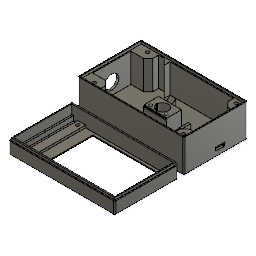
Wärmebildkamera-Gehäuse-v49 (Autodesk Fusion 360 design; units mm, degrees)
Autodesk Fusion 360 part; units mm, degrees
box "Grundkörper Quader1" add length 55 width 92 height 11 placed x (0, 0, 1) y (1, 0, 0) z (0, 1, 0) at (-92, 0, 0) makes body 1
box "Grundkörper Quader3" cut length 51 width 83 height -6 placed x (0, 0, -1) y (-1, 0, 0) z (0, 1, 0) at (-2, 11, 53) bodies 1
box "Grundkörper Quader4" cut length 45.9499 width 60 height -6 placed x (0, 0, -1) y (-1, 0, 0) z (0, 1, 0) at (-9.4927, 5, 50.5086) bodies 1
box "Grundkörper Quader5" cut length 51 width 82 height -4 placed x (0, 0, -1) y (-1, 0, 0) z (0, 1, 0) at (-8, 5, 53) bodies 1
sketch "Skizze11" plane through (0, 11, 0) normal (0, 1, 0) x (-1, 0, 0)
  line L0 (2, 53) -> (85, 53)
  line L1 (85, 53) -> (85, 2)
  line L2 (85, 2) -> (2, 2)
  line L3 (2, 2) -> (2, 53)
  line L4 (0, 0) -> (92, 0)
  line L5 (92, 0) -> (92, 55)
  line L6 (92, 55) -> (0, 55)
  line L7 (0, 55) -> (0, 0)
  line L8 (85, 53) -> (90, 53)
  line L9 (90, 53) -> (90, 2)
  line L10 (90, 2) -> (85, 2)
  line L11 (85, 2) -> (85, 53)
extrude "Extrusion1" cut sketch "Skizze11" against normal blind 4 contours L1 L8 L9 L10 L11 bodies 1
sketch "Skizze15" plane through (0, 11, 0) normal (0, 1, 0) x (-1, 0, 0)
  line L0 (2, 53) -> (90, 53)
  line L1 (90, 53) -> (90, 2)
  line L2 (90, 2) -> (2, 2)
  line L3 (2, 2) -> (2, 53)
  line L4 (0, 0) -> (92, 0)
  line L5 (92, 0) -> (92, 55)
  line L6 (92, 55) -> (0, 55)
  line L7 (0, 55) -> (0, 0)
  line L8 (91, 1) -> (1, 1)
  line L9 (1, 1) -> (1, 54)
  line L10 (1, 54) -> (91, 54)
  line L11 (91, 54) -> (91, 1)
extrude "Extrusion3" add sketch "Skizze15" along normal blind 2 contours L8 L9 L10 L11 bodies 1
sketch "Skizze16" plane through (0, 0, 0) normal (0, 1, 0) x (1, 0, 0)
  line L0 (0, 5) -> (-92, 5)
  line L1 (-92, 5) -> (-92, 60)
  line L2 (-92, 60) -> (0, 60)
  line L3 (0, 60) -> (0, 5)
extrude "Extrusion4" add sketch "Skizze16" along normal blind 2 separate body makes body 2
sketch "Skizze17" plane through (0, 2, 0) normal (0, 1, 0) x (-1, 0, 0)
  line L0 (0, -60) -> (92, -60)
  line L1 (92, -60) -> (92, -5)
  line L2 (92, -5) -> (0, -5)
  line L3 (0, -5) -> (0, -60)
  line L4 (90, -58) -> (2, -58)
  line L5 (2, -58) -> (2, -7)
  line L6 (2, -7) -> (90, -7)
  line L7 (90, -7) -> (90, -58)
extrude "Extrusion5" add sketch "Skizze17" along normal blind 25 bodies 2
sketch "Skizze18" plane through (0, 27, 0) normal (0, 1, 0) x (-1, 0, 0)
  line L0 (2, -7) -> (90, -7)
  line L1 (90, -7) -> (90, -58)
  line L2 (90, -58) -> (2, -58)
  line L3 (2, -58) -> (2, -7)
  line L4 (0, -5) -> (0, -60)
  line L5 (0, -60) -> (92, -60)
  line L6 (92, -60) -> (92, -5)
  line L7 (92, -5) -> (0, -5)
  line L8 (91, -59) -> (1, -59)
  line L9 (1, -59) -> (1, -6)
  line L10 (1, -6) -> (91, -6)
  line L11 (91, -6) -> (91, -59)
extrude "Extrusion6" add sketch "Skizze18" along normal blind 2 contours L4 L5 L6 L7 bodies 2
sketch "Skizze19" plane through (0, 2, 0) normal (0, 1, 0) x (-1, 0, 0)
  line L0 (2, -7) -> (2, -58)
  line L1 (2, -58) -> (90, -58)
  line L2 (90, -58) -> (90, -7)
  line L3 (90, -7) -> (2, -7)
  line L4 (10, -7) -> (75, -7)
  line L5 (75, -7) -> (75, -26.5)
  line L6 (75, -26.5) -> (10, -26.5)
  line L7 (10, -26.5) -> (10, -7)
  dimension "d50" = 65
  dimension "d51" = 19.5
extrude "Extrusion7" add sketch "Skizze19" along normal blind 12 contours L3 L4 L5 L6 L7 bodies 2
sketch "Skizze20" plane through (-75, 0, 0) normal (-1, 0, 0) x (0, 0, 1)
  line L0 (-26.5, 2) -> (-7, 2)
  line L1 (-7, 2) -> (-7, 14)
  line L2 (-7, 14) -> (-26.5, 14)
  line L3 (-26.5, 14) -> (-26.5, 2)
  circle A0 centre (-16.75, 11.25) radius 9.25
  dimension "d54" = 18.5
  measures "d54" diameter of A0
extrude "Extrusion8" cut sketch "Skizze20" against normal blind 65 contours L2 A0 picked at (-17.65, 9.3946) bodies 2
sketch "Skizze21" plane through (0, 2, 0) normal (0, 1, 0) x (-1, 0, 0)
  line L0 (75, -7) -> (75, -16.75)
  line L1 (75, -16.75) -> (75, -26.5)
  line L2 (75, -26.5) -> (10, -26.5)
  line L3 (10, -26.5) -> (10, -16.75)
  line L4 (10, -16.75) -> (10, -7)
  line L5 (10, -7) -> (2, -7)
  line L6 (2, -7) -> (2, -58)
  line L7 (2, -58) -> (90, -58)
  line L8 (90, -58) -> (90, -7)
  line L9 (90, -7) -> (75, -7)
  circle A0 centre (46, -32.5) radius 4.75
  line L10 (56.0142, -26.5) -> (36, -26.5)
  line L11 (36, -26.5) -> (36, -39)
  line L12 (36, -39) -> (56.0142, -39)
  line L13 (56.0142, -39) -> (56.0142, -26.5)
  dimension "d57" = 9.5
  measures "d57" diameter of A0
extrude "Extrusion9" add sketch "Skizze21" along normal blind 13 contours L2 L10 L11 L12 L13 bodies 2
extrude "Extrusion10" cut 1 faces at (-47.2238, 2, -31.2621) along direction (0, -1, 0) blind 2 on bodies 2 bodies 2
sketch "Skizze22" plane through (0, 15, 0) normal (0, 1, 0) x (-1, 0, 0)
  circle A0 centre (46, -32.5) radius 4.75
  line L0 (56.0142, -39) -> (56.0142, -26.5)
  line L1 (56.0142, -26.5) -> (36, -26.5)
  line L2 (36, -26.5) -> (36, -39)
  line L3 (36, -39) -> (56.0142, -39)
  line L4 (51.5, -33) -> (50.5, -33)
  line L5 (50.5, -33) -> (50.5, -32)
  line L6 (50.5, -32) -> (51.5, -32)
  line L7 (51.5, -32) -> (51.5, -33)
extrude "Extrusion11" cut sketch "Skizze22" against normal blind 5 contours A0 L4 L6 L7 bodies 2
sketch "Skizze24" plane through (0, 2, 0) normal (0, 1, 0) x (-1, 0, 0)
  line L0 (56.0142, -26.5) -> (56.0142, -39)
  line L1 (56.0142, -39) -> (36, -39)
  line L2 (36, -39) -> (36, -26.5)
  line L3 (36, -26.5) -> (10, -26.5)
  line L4 (10, -26.5) -> (10, -16.75)
  line L5 (10, -16.75) -> (10, -7)
  line L6 (10, -7) -> (2, -7)
  line L7 (2, -7) -> (2, -58)
  line L8 (2, -58) -> (90, -58)
  line L9 (90, -58) -> (90, -7)
  line L10 (90, -7) -> (75, -7)
  line L11 (75, -7) -> (75, -16.75)
  line L12 (75, -16.75) -> (75, -26.5)
  line L13 (75, -26.5) -> (56.0142, -26.5)
  line L14 (82, -58) -> (90, -58)
  line L15 (90, -58) -> (90, -49)
  line L16 (90, -49) -> (82, -49)
  line L17 (82, -49) -> (82, -58)
  line L18 (90, -16) -> (82, -16)
  line L19 (82, -16) -> (82, -7)
  line L20 (82, -7) -> (90, -7)
  line L21 (90, -7) -> (90, -16)
  line L22 (2, -58) -> (10, -58)
  line L23 (10, -58) -> (10, -49)
  line L24 (10, -49) -> (2, -49)
  line L25 (2, -49) -> (2, -58)
  line L26 (2, -7) -> (10, -7)
  line L27 (10, -7) -> (10, -16)
  line L28 (10, -16) -> (2, -16)
  line L29 (2, -16) -> (2, -7)
extrude "Extrusion13" add sketch "Skizze24" along normal blind 27 contours L9 L10 L18 L19 L20 L21 | L5 L6 L7 L26 L27 L28 L29 | L8 L9 L14 L15 L16 L17 | L7 L8 L22 L23 L24 L25 bodies 2
sketch "Skizze25" plane through (0, 29, 0) normal (0, 1, 0) x (-1, 0, 0)
  line L0 (90, -7) -> (82, -7)
  line L1 (82, -7) -> (82, -16)
  line L2 (82, -16) -> (90, -16)
  line L3 (90, -16) -> (90, -7)
  circle A0 centre (5, -55.5) radius 1.5
  circle A1 centre (5, -9.5) radius 1.5
  dimension "d72" = 3
  dimension "d73" = 3
  measures "d72" diameter of A0
  measures "d73" diameter of A1
extrude "Extrusion14" cut sketch "Skizze25" against normal blind 25 contours A0 | A1 bodies 2
extrude "Extrusion15" cut 4 faces at (-84.6667, 29, -52) (-84.6667, 29, -10) (-5.7779, 29, -14.3208) (-5.7779, 29, -50.6792) along direction (0, -1, 0) blind 7 on bodies 2 bodies 2
delete_face "Fläche löschen1" 1 faces at (-50.6361, 8.3333, -33.5338) on bodies 2
sketch "Skizze26" plane through (0, 15, 0) normal (0, 1, 0) x (-1, 0, 0)
  line L0 (36, -26.5) -> (36, -39)
  line L1 (36, -39) -> (56.0142, -39)
  line L2 (56.0142, -39) -> (56.0142, -26.5)
  line L3 (56.0142, -26.5) -> (36, -26.5)
  circle A0 centre (46.0071, -32.5) radius 5
  circle A1 centre (39.2493, -29) radius 1.5
  circle A2 centre (52.7493, -29) radius 1.5
  line L4 (51.5, -33) -> (50.9821, -33)
  line L5 (51.5, -33) -> (51.5, -32)
  line L6 (51.5, -32) -> (50.9821, -32)
  line L7 (46.0088, -27.5) -> (52.7588, -27.5022)
  dimension "d78" = 10
  dimension "d81" = 3
  dimension "d82" = 3
  dimension "d87" = 6.75
  measures "d78" diameter of A0
  measures "d81" diameter of A1
  measures "d82" diameter of A2
extrude "Extrusion16" cut sketch "Skizze26" against normal blind 15 contours A0 bodies 2
extrude "Extrusion17" cut sketch "Skizze26" against normal blind 13 contours A1 | A2 bodies 2
thread "Gewinde5" "ISO Metric profile 3.0 M3x0.5 6H" major diameter 3.086 minor diameter 2.529 pitch 0.5 angle 60 resizes the face on face at (-52.1324, 6.3333, -30.3673) on bodies 2
thread "Gewinde6" "ISO Metric profile 3.0 M3x0.5 6H" major diameter 3.086 minor diameter 2.529 pitch 0.5 angle 60 resizes the face on face at (-38.565, 10.6667, -30.3348) on bodies 2
move_face "Fläche verschieben1" by (-1, 0, 0) 1 faces at (-9.4927, 0.3333, 35.1919) on bodies 1
extrude "Extrusion18" cut sketch "Skizze26" against normal blind 6 contours A0 L4 L5 L6 bodies 2
fillet "Abrundung1" radius 1 1 edges at (0, 14.5, -60) on bodies 2
fillet "Abrundung2" radius 1 1 edges at (0, 14.5, -5) on bodies 2
fillet "Abrundung3" radius 1 5 edges at (-46.5, 0, -60) (-0.2929, 0, -59.7071) (0, 0, -32.5) (-0.2929, 0, -5.2929) (-46.5, 0, -5) on bodies 2
fillet "Abrundung4" radius 1 5 edges at (-92, 15, -5) (-92, 0.2929, -5.2929) (-92, 0, -32.5) (-92, 0.2929, -59.7071) (-92, 15, -60) on bodies 2
fillet "Abrundung5" radius 1 1 edges at (0, 0, 27.5) on bodies 1
fillet "Abrundung6" radius 1 3 edges at (0, 6, 55) (-0.2929, 0.2929, 55) (-46.5, 0, 55) on bodies 1
fillet "Abrundung7" radius 1 3 edges at (0, 6, 0) (-0.2929, 0.2929, 0) (-46.5, 0, 0) on bodies 1
fillet "Abrundung8" radius 1 5 edges at (-92, 6, 55) (-92, 0.2929, 54.7071) (-92, 0, 27.5) (-92, 0.2929, 0.2929) (-92, 6, 0) on bodies 1
sketch "Skizze27" plane through (0, 2, 0) normal (0, 1, 0) x (-1, 0, 0)
  line L0 (82, -58) -> (82, -49)
  line L1 (82, -49) -> (90, -49)
  line L2 (90, -49) -> (90, -16)
  line L3 (90, -16) -> (82, -16)
  line L4 (82, -16) -> (82, -7)
  line L5 (82, -7) -> (75, -7)
  line L6 (75, -7) -> (75, -16.75)
  line L7 (75, -16.75) -> (75, -26.5)
  line L8 (75, -26.5) -> (56.0142, -26.5)
  line L9 (56.0142, -26.5) -> (56.0142, -39)
  line L10 (56.0142, -39) -> (36, -39)
  line L11 (36, -39) -> (36, -26.5)
  line L12 (36, -26.5) -> (10, -26.5)
  line L13 (10, -26.5) -> (10, -16.75)
  line L14 (10, -16.75) -> (10, -16)
  line L15 (10, -16) -> (2, -16)
  line L16 (2, -16) -> (2, -49)
  line L17 (2, -49) -> (10, -49)
  line L18 (10, -49) -> (10, -58)
  line L19 (10, -58) -> (82, -58)
  line L20 (2, -28) -> (28, -28)
  line L21 (28, -28) -> (28, -45)
  line L22 (28, -45) -> (2, -45)
  line L23 (2, -45) -> (2, -28)
  line L24 (7, -44) -> (23, -44)
  line L25 (23, -44) -> (23, -48)
  line L26 (23, -48) -> (7, -48)
  line L27 (7, -48) -> (7, -44)
  line L28 (7, -29) -> (23, -29)
  line L29 (23, -29) -> (23, -26.5)
  line L30 (23, -26.5) -> (7, -26.5)
  line L31 (7, -26.5) -> (7, -29)
  dimension "d98" = 26
  dimension "d99" = 17
  measures "d98" distance of origin
extrude "Extrusion19" add sketch "Skizze27" along normal blind 5 contours L22 L24 L25 L27 | L22 L25 L26 L27 | L12 L20 L29 L30 L31 | L20 L28 L29 L31 bodies 2
sketch "Skizze28" plane through (-23, 0, 0) normal (-1, 0, 0) x (0, 0, 1)
  line L0 (-48, 2) -> (-44, 2)
  line L1 (-44, 2) -> (-44, 7)
  line L2 (-44, 7) -> (-48, 7)
  line L3 (-48, 7) -> (-48, 2)
  line L4 (-44, 4) -> (-45.3671, 4)
  line L5 (-45.3671, 4) -> (-45.3671, 22.3058)
  line L6 (-45.3671, 22.3058) -> (-45.3907, 7)
  line L7 (-45.4065, 7) -> (-45.3907, 7)
  line L8 (-46, 7) -> (-48, 2)
  line L9 (-29, 2) -> (-29, 7)
  line L10 (-29, 4) -> (-28, 4)
  line L11 (-28, 4) -> (-28, 5)
  line L12 (-28, 5) -> (-29, 6)
  line L13 (-26.5, 7) -> (-29, 7)
  line L14 (-29, 6) -> (-28, 7)
extrude "Extrusion20" cut sketch "Skizze28" against normal blind 17 contours L2 L3 L8 | L1 L2 L4 L5 | L9 L10 L11 L12 bodies 2
sketch "Skizze29" plane through (-2, 0, 0) normal (-1, 0, 0) x (0, 0, 1)
  line L0 (-49, 22) -> (-49, 2)
  line L1 (-49, 2) -> (-16, 2)
  line L2 (-16, 2) -> (-16, 22)
  line L3 (-16, 22) -> (-7, 22)
  line L4 (-45.3671, 4) -> (-28, 4)
  line L5 (-28, 4) -> (-28, 5)
  line L6 (-28, 5) -> (-45.3671, 5)
  line L7 (-45.3671, 5) -> (-45.3671, 4)
  line L8 (-36.6835, 5) -> (-32.5, 5)
  line L9 (-32.5, 5) -> (-32.5, 8)
  line L10 (-32.5, 8) -> (-36.6835, 8)
  line L11 (-36.6835, 8) -> (-36.6835, 5)
  line L12 (-32.5, 8) -> (-40.5, 8)
  line L13 (-40.5, 8) -> (-40.5, 5)
  line L14 (-40.5, 5) -> (-32.5, 5)
  line L15 (-32.5, 5) -> (-32.5, 8)
  line L16 (-7, 22) -> (-7, 27)
  line L17 (-7, 27) -> (-58, 27)
  line L18 (-58, 27) -> (-58, 22)
  line L19 (-58, 22) -> (-49, 22)
extrude "Extrusion21" cut sketch "Skizze29" against normal blind 11 contours L6 L11 L12 L13 L14 | L6 L8 L9 L10 L11 L12 L14 L15 bodies 2
sketch "Skizze30" plane through (0, 2, 0) normal (0, 1, 0) x (-1, 0, 0)
  line L0 (23, -26.5) -> (23, -29)
  line L1 (23, -29) -> (7, -29)
  line L2 (7, -29) -> (7, -26.5)
  line L3 (10, -16.75) -> (10, -16)
  line L4 (10, -16) -> (2, -16)
  line L5 (2, -16) -> (2, -49)
  line L6 (2, -49) -> (10, -49)
  line L7 (10, -49) -> (10, -58)
  line L8 (10, -58) -> (82, -58)
  line L9 (82, -58) -> (82, -49)
  line L10 (82, -49) -> (90, -49)
  line L11 (90, -49) -> (90, -16)
  line L12 (90, -16) -> (82, -16)
  line L13 (82, -16) -> (82, -7)
  line L14 (82, -7) -> (75, -7)
  line L15 (75, -7) -> (75, -16.75)
  line L16 (75, -16.75) -> (75, -26.5)
  line L17 (75, -26.5) -> (56.0142, -26.5)
  line L18 (56.0142, -26.5) -> (56.0142, -39)
  line L19 (56.0142, -39) -> (36, -39)
  line L20 (36, -39) -> (36, -26.5)
  line L21 (36, -26.5) -> (23, -26.5)
  line L22 (7, -48) -> (7, -44)
  line L23 (7, -44) -> (23, -44)
  line L24 (23, -44) -> (23, -48)
  line L25 (23, -48) -> (7, -48)
  line L26 (2, -32.5) -> (2, -40.5)
  line L27 (2, -36.5) -> (28.5, -36.5)
  line L28 (29.5, -40.4445) -> (33.5, -40.4445)
  line L29 (33.5, -40.4445) -> (33.5, -32.4445)
  line L30 (33.5, -32.4445) -> (29.5, -32.4445)
  line L31 (29.5, -32.4445) -> (29.5, -40.4445)
  line L32 (7, -26.5) -> (10, -26.5)
  line L33 (10, -26.5) -> (10, -16.75)
  dimension "d107" = 26.5
  measures "d107" distance of origin
extrude "Extrusion22" add sketch "Skizze30" along normal blind 5 contours L28 L29 L30 L31 bodies 2
sketch "Skizze31" plane through (0, 0, -26.5) normal (0, 0, -1) x (-1, 0, 0)
  line L0 (10, 7) -> (23, 7)
  line L1 (23, 7) -> (23, 2)
  line L2 (23, 2) -> (36, 2)
  line L3 (36, 2) -> (36, 14)
  line L4 (36, 14) -> (10, 14)
  line L5 (10, 14) -> (10, 7)
  line L6 (10, 7) -> (36, 7)
  line L7 (36, 7) -> (36, 14)
  line L8 (36, 14) -> (10, 14)
  line L9 (10, 14) -> (10, 7)
  line L10 (56.0142, 7) -> (75, 7)
  line L11 (75, 7) -> (75, 14)
  line L12 (75, 14) -> (56.0142, 14)
  line L13 (56.0142, 14) -> (56.0142, 7)
  line L14 (56.0142, 14) -> (56.0142, 2)
extrude "Extrusion23" cut sketch "Skizze31" against normal blind 4 contours L0 L3 L4 L5 L6 L7 L8 L9 | L10 L11 L12 L13 L14 bodies 2
sketch "Skizze32" plane through (0, 2, 0) normal (0, 1, 0) x (-1, 0, 0)
  line L0 (29.5, -32.4445) -> (33.5, -32.4445)
  line L1 (33.5, -32.4445) -> (33.5, -40.4445)
  line L2 (33.5, -40.4445) -> (29.5, -40.4445)
  line L3 (29.5, -40.4445) -> (29.5, -32.4445)
  line L4 (23, -26.5) -> (23, -29)
  line L5 (23, -29) -> (7, -29)
  line L6 (7, -29) -> (7, -26.5)
  line L7 (10, -16.75) -> (10, -16)
  line L8 (10, -16) -> (2, -16)
  line L9 (2, -16) -> (2, -49)
  line L10 (2, -49) -> (10, -49)
  line L11 (10, -49) -> (10, -58)
  line L12 (10, -58) -> (82, -58)
  line L13 (82, -58) -> (82, -49)
  line L14 (82, -49) -> (90, -49)
  line L15 (90, -49) -> (90, -16)
  line L16 (90, -16) -> (82, -16)
  line L17 (82, -16) -> (82, -7)
  line L18 (82, -7) -> (75, -7)
  line L19 (75, -7) -> (75, -16.75)
  line L20 (75, -16.75) -> (75, -26.5)
  line L21 (75, -26.5) -> (56.0142, -26.5)
  line L22 (56.0142, -26.5) -> (56.0142, -39)
  line L23 (56.0142, -39) -> (36, -39)
  line L24 (36, -39) -> (36, -26.5)
  line L25 (36, -26.5) -> (23, -26.5)
  line L26 (7, -48) -> (7, -44)
  line L27 (7, -44) -> (23, -44)
  line L28 (23, -44) -> (23, -48)
  line L29 (23, -48) -> (7, -48)
  line L30 (36, -39) -> (56, -39)
  line L31 (56, -39) -> (56, -39.7497)
  line L32 (56, -39.7497) -> (36, -39.7497)
  line L33 (36, -39.7497) -> (36, -39)
  line L34 (36, -58) -> (56, -58)
  line L35 (56, -58) -> (56, -56)
  line L36 (56, -56) -> (36, -56)
  line L37 (36, -56) -> (36, -58)
  line L38 (7, -26.5) -> (10, -26.5)
  line L39 (10, -26.5) -> (10, -16.75)
sketch "Skizze34" plane through (0, 0, -40.4445) normal (0, 0, -1) x (-1, 0, 0)
  line L0 (29.5, 2) -> (33.5, 2)
  line L1 (33.5, 2) -> (33.5, 7)
  line L2 (33.5, 7) -> (29.5, 7)
  line L3 (29.5, 7) -> (29.5, 2)
  line L4 (33.5, 2) -> (31.5, 7)
extrude "Extrusion27" cut sketch "Skizze34" against normal blind 9 contours L1 L2 L4 bodies 2
sketch "Skizze35" plane through (-92, 0, 0) normal (-1, 0, 0) x (0, 0, 1)
  line L0 (-6, 1) -> (-6, 29)
  line L1 (-6, 29) -> (-59, 29)
  line L2 (-59, 29) -> (-59, 1)
  line L3 (-59, 1) -> (-6, 1)
  circle A0 centre (-32.5, 12) radius 6
  dimension "d120" = 12
  measures "d120" diameter of A0
extrude "Extrusion28" cut sketch "Skizze35" against normal blind 30 contours A0 bodies 2
sketch "Skizze38" plane through (0, 27, 0) normal (0, 1, 0) x (-1, 0, 0)
  line L0 (1, -6) -> (1, -59)
  line L1 (1, -59) -> (91, -59)
  line L2 (91, -59) -> (91, -6)
  line L3 (91, -6) -> (1, -6)
  line L4 (2, -7) -> (90, -7)
  line L5 (90, -7) -> (90, -58)
  line L6 (90, -58) -> (2, -58)
  line L7 (2, -58) -> (2, -7)
chamfer "Fase2" distance 0.5 angle 45 1 edges at (-1, 5, -40.5) on bodies 2
chamfer "Fase3" distance 0.5 angle 45 1 edges at (-1, 5, -32.5) on bodies 2
extrude "Extrusion31" add 2 faces at (-31.6667, 9.6667, 2) (-88.3333, 9.6667, 2) along direction (0, 0, 1) blind 0.75 on bodies 1 bodies 1
extrude "Extrusion32" add 1 faces at (-31.6667, 8.3333, 53) along direction (0, 0, -1) blind 0.75 on bodies 1 bodies 1
extrude "Extrusion33" cut 1 faces at (-86.6667, 7, 19.25) along direction (0, -1, 0) blind 2 on bodies 1 bodies 1
extrude "Extrusion34" add 1 faces at (-8, 2.3333, 35.75) along direction (-1, 0, 0) blind 0.5 on bodies 1 bodies 1
sketch "Skizze40" plane through (0, 5, 0) normal (0, 1, 0) x (-1, 0, 0)
  line L0 (8.5, 52.25) -> (2, 52.25)
  line L1 (2, 52.25) -> (2, 2.75)
  line L2 (2, 2.75) -> (8.5, 2.75)
  line L3 (8.5, 2.75) -> (8.5, 52.25)
  circle A0 centre (5, 5.5) radius 1.5
  circle A1 centre (5, 49.5) radius 1.5
  dimension "d149" = 3
  dimension "d150" = 3
  measures "d149" diameter of A0
  measures "d150" diameter of A1
extrude "Extrusion35" cut sketch "Skizze40" against normal blind 26 contours A0 | A1 bodies 1
sketch "Skizze45" plane through (0, 1, 0) normal (0, 1, 0) x (-1, 0, 0)
  line L0 (8.5, 52.25) -> (8.5, 2.75)
  line L1 (8.5, 2.75) -> (90, 2.75)
  line L2 (90, 2.75) -> (90, 52.25)
  line L3 (90, 52.25) -> (8.5, 52.25)
  line L4 (69.4927, 50.5086) -> (69.4927, 4.5586)
  line L5 (69.4927, 4.5586) -> (10.4927, 4.5586)
  line L6 (10.4927, 4.5586) -> (10.4927, 50.5086)
  line L7 (10.4927, 50.5086) -> (69.4927, 50.5086)
  line L8 (90, 2.75) -> (78.5, 2.75)
  line L9 (78.5, 2.75) -> (78.5, 52.25)
  line L10 (78.5, 52.25) -> (90, 52.25)
  line L11 (90, 52.25) -> (90, 2.75)
  line L12 (78.5, 2.75) -> (85.5, 2.75)
  line L13 (85.5, 2.75) -> (85.5, 52.25)
  line L14 (85.5, 52.25) -> (78.5, 52.25)
  line L15 (78.5, 52.25) -> (78.5, 2.75)
extrude "Extrusion36" add sketch "Skizze45" along normal blind 2 contours L1 L3 L8 L9 L10 L12 L13 L14 L15 bodies 1
extrude "Extrusion37" cut 1 faces at (-7.7838, 5, 20.3836) along direction (0, -1, 0) blind 2 on bodies 1 bodies 1
sketch "Skizze46" plane through (0, 3, 0) normal (0, 1, 0) x (-1, 0, 0)
  line L0 (78.5, 52.25) -> (78.5, 2.75)
  line L1 (78.5, 2.75) -> (85.5, 2.75)
  line L2 (85.5, 2.75) -> (85.5, 52.25)
  line L3 (85.5, 52.25) -> (78.5, 52.25)
  circle A0 centre (82, 5.5) radius 1.5
  circle A1 centre (82, 49.4987) radius 1.5
  dimension "d159" = 3
  dimension "d160" = 3
  measures "d159" diameter of A0
  measures "d160" diameter of A1
extrude "Extrusion38" cut sketch "Skizze46" against normal blind 10 contours A0 | A1 bodies 1
extrude "Extrusion39" add 2 faces at (-82, 8.6667, -13) (-82, 15.3333, -52) along direction (1, 0, 0) blind 7 on bodies 2 bodies 2
sketch "Skizze47" plane through (0, 27, 0) normal (0, 1, 0) x (-1, 0, 0)
  line L0 (1, -6) -> (1, -59)
  line L1 (1, -59) -> (91, -59)
  line L2 (91, -59) -> (91, -6)
  line L3 (91, -6) -> (1, -6)
  line L4 (2, -7) -> (90, -7)
  line L5 (90, -7) -> (90, -58)
  line L6 (90, -58) -> (2, -58)
  line L7 (2, -58) -> (2, -7)
  circle A0 centre (82, -55.5) radius 1.5
  circle A1 centre (82, -9.5) radius 1.5
  dimension "d165" = 3
  dimension "d166" = 3
  measures "d165" diameter of A0
  measures "d166" diameter of A1
extrude "Extrusion40" add 4 faces at (-85, 22, -13) (-80, 22, -55) (-5.7779, 22, -50.6792) (-5.7779, 22, -14.3208) along direction (0, 1, 0) blind 5 on bodies 2 bodies 2
extrude "Extrusion41" cut sketch "Skizze47" against normal blind 23 contours A0 | A1 bodies 2
sketch "Skizze48" plane through (0, 2, 0) normal (0, 1, 0) x (-1, 0, 0)
  line L0 (75, -49) -> (90, -49)
  line L1 (90, -49) -> (90, -16)
  line L2 (90, -16) -> (75, -16)
  line L3 (75, -16) -> (75, -16.75)
  line L4 (75, -16.75) -> (75, -26.5)
  line L5 (75, -26.5) -> (56.0142, -26.5)
  line L6 (56.0142, -26.5) -> (56.0142, -39)
  line L7 (56.0142, -39) -> (36, -39)
  line L8 (36, -39) -> (36, -26.5)
  line L9 (36, -26.5) -> (23, -26.5)
  line L10 (23, -26.5) -> (23, -29)
  line L11 (23, -29) -> (7, -29)
  line L12 (7, -29) -> (7, -26.5)
  line L13 (7, -26.5) -> (10, -26.5)
  line L14 (10, -26.5) -> (10, -16.75)
  line L15 (10, -16.75) -> (10, -16)
  line L16 (10, -16) -> (2, -16)
  line L17 (2, -16) -> (2, -49)
  line L18 (2, -49) -> (10, -49)
  line L19 (10, -49) -> (10, -58)
  line L20 (10, -58) -> (75, -58)
  line L21 (75, -58) -> (75, -49)
  line L22 (29.5, -32.4445) -> (33.5, -32.4445)
  line L23 (33.5, -32.4445) -> (33.5, -40.4445)
  line L24 (33.5, -40.4445) -> (29.5, -40.4445)
  line L25 (29.5, -40.4445) -> (29.5, -32.4445)
  line L26 (7, -48) -> (7, -44)
  line L27 (7, -44) -> (23, -44)
  line L28 (23, -44) -> (23, -48)
  line L29 (23, -48) -> (7, -48)
  line L30 (10, -58) -> (65, -58)
  line L31 (65, -58) -> (65, -53)
  line L32 (65, -53) -> (10, -53)
  line L33 (10, -53) -> (10, -58)
  line L34 (65, -53) -> (70, -53)
  line L35 (70, -53) -> (70, -58)
  line L36 (70, -58) -> (65, -58)
  line L37 (65, -58) -> (65, -53)
  line L38 (60, -48) -> (55, -48)
  line L39 (55, -48) -> (55, -53)
  line L40 (55, -53) -> (60, -53)
  line L41 (60, -53) -> (60, -48)
  line L42 (15, -48) -> (20, -48)
  line L43 (20, -48) -> (20, -53)
  line L44 (20, -53) -> (15, -53)
  line L45 (15, -53) -> (15, -48)
  dimension "d171" = 55
  dimension "d172" = 5
  dimension "d173" = 5
  measures "d171" distance of origin
  measures "d173" distance of origin
extrude "Extrusion42" add sketch "Skizze48" along normal blind 25 contours L20 L31 L34 L35 L36 L37 bodies 2
extrude "Extrusion43" add sketch "Skizze48" along normal blind 5 contours L32 L38 L39 L40 L41 | L29 L32 L42 L43 L44 L45 bodies 2
chamfer "Fase4" distance 5 angle 45 1 edges at (-57.5, 7, -48) on bodies 2
chamfer "Fase5" distance 5 angle 45 1 edges at (-70, 14.5, -53) on bodies 2
chamfer "Fase6" distance 5 angle 45 1 edges at (-17.5, 7, -48) on bodies 2
chamfer "Fase7" distance 4 angle 45 1 edges at (-75, 14.5, -49) on bodies 2
chamfer "Fase8" distance 4 angle 45 1 edges at (-75, 14.5152, -16) on bodies 2
chamfer "Fase9" distance 4 angle 45 1 edges at (-10, 14.5152, -16) on bodies 2
chamfer "Fase10" distance 4 angle 45 1 edges at (-10, 14.5, -49) on bodies 2
extrude "Extrusion44" cut 1 faces at (-56.8333, 9.6667, 52.25) along direction (0, 0, 1) blind 0.5 on bodies 1 bodies 1
extrude "Extrusion45" cut 2 faces at (-29.6667, 6.3333, 2.75) (-88.3333, 9, 2.75) along direction (0, 0, -1) blind 0.5 on bodies 1 bodies 1
sketch "Skizze49" plane through (0, 1, 0) normal (0, 1, 0) x (-1, 0, 0)
  line L0 (85.5, 52.75) -> (85.5, 2.25)
  line L1 (85.5, 2.25) -> (90, 2.25)
  line L2 (90, 2.25) -> (90, 52.75)
  line L3 (90, 52.75) -> (85.5, 52.75)
  line L4 (90, 2.25) -> (89, 2.25)
  line L5 (89, 2.25) -> (89, 52.75)
  line L6 (89, 52.75) -> (90, 52.75)
  line L7 (90, 52.75) -> (90, 2.25)
  dimension "d189" = 1
extrude "Extrusion46" add sketch "Skizze49" along normal blind 2 contours L1 L2 L3 L4 L5 L6 L7 bodies 1
extrude "Extrusion47" add 1 faces at (-89.3333, 3, 35.9167) along direction (0, 1, 0) blind 2 on bodies 1 bodies 1
move_face "Fläche verschieben2" to x (1, 0, 0) y (0, 1, 0) z (0, 0, 1) at (0.5, 0, 0) 5 faces at (-80.8509, 1, 6.4642) (-84.7838, 3, 34.6159) (-85.5, 2.3333, 35.9167) (-80.8043, 1, 48.593) (-78.5, 2.3333, 35.9167) on bodies 1
extrude "Extrusion48" add 1 faces at (-89, 3.6667, 35.9167) along direction (1, 0, 0) blind 0.5 on bodies 1 bodies 1
sketch "Skizze50" plane through (0, 0, 0) normal (0, 1, 0) x (1, 0, 0)
sketch "Skizze51" plane through (0, 0, 0) normal (0, 1, 0) x (1, 0, 0)
